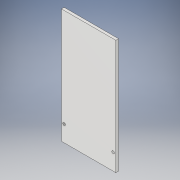
# Autodesk Inventor part: Part12
Saved by Autodesk Inventor 2017 SP1 (Build 210196100, 196)
## iProperties
Created: 2017-05-14
Part Number: Part12
Material: ABS Plastic
Document SubType Name: Modeling
Designer: Zach
Density: 1.06 g/cm^3
Appearance: Smooth - White
Author: Zach
Autodesk Inventor part; units mm, degrees
ref_plane "YZ Plane" through (0, 0, 0) normal (1, 0, 0) x (0, 1, 0)
ref_plane "XZ Plane" through (0, 0, 0) normal (0, 1, 0) x (-1, 0, 0)
ref_plane "XY Plane" through (0, 0, 0) normal (0, 0, 1) x (1, 0, 0)
sketch "Sketch1" plane through (0, 0, 0) normal (0, 0, 1) x (1, 0, 0)
  line L0 (0, 0) -> (100, 0)
  line L1 (100, 0) -> (100, 210.727)
  line L2 (100, 210.727) -> (0, 210.727)
  line L3 (0, 210.727) -> (0, 0)
  dimension "d0" = 100
  dimension "d1" = 210.7269
  constraints: 8 end point, 2 parallel, 1 horizontal, 1 perpendicular
  measures "d0" distance of L2.end L1.end
  measures "d1" distance of L1.end L0.end
extrude "Extrusion1" add sketch "Sketch1" along normal blind 5
sketch "Sketch2" plane through (0, 0, 5) normal (0, 0, 1) x (1, 0, 0)
  circle A0 centre (5, 29.9257) radius 2.5
  circle A1 centre (95, 29.9257) radius 2.5
  line L0 (100, 0) -> (100, 210.727) projected
  line L1 (0, 0) -> (100, 0) projected
  dimension "d4" = 5
  dimension "d5" = 5
  dimension "d6" = 95
  dimension "d7" = 5
  dimension "d8" = 29.9257
  dimension "d9" = 29.9257
  constraints: 2 centre point
  measures "d4" diameter of A0
  measures "d5" diameter of A1
  measures "d6" distance from line of L0 A0.centre
  measures "d7" distance from line of L0 A1.centre
  measures "d8" distance from line of L1 A0.centre
  measures "d9" distance from line of L1 A1.centre
extrude "Extrusion2" cut sketch "Sketch2" against normal blind 5
body "Solid1"
